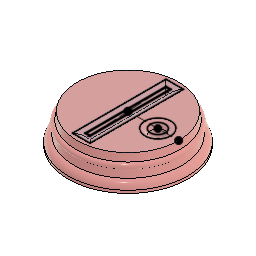
SoilSensorWaterProofCap (Autodesk Fusion 360 design; units mm, degrees)
Autodesk Fusion 360 part; units mm, degrees
note: some values were not read from the file. Set by a fixed rule: which face or edge a step refers to.
sketch "Sketch1" plane through (0, 0, 0) normal (0, 0, 1) x (1, 0, 0) in component "Cap"
  circle A0 centre (0, 0) radius 16.5
  circle A1 centre (0, 0) radius 14.9
  dimension "d1" = 33
  dimension "d2" = 29.8
  constraint coincident A0.centre A1.centre
  constraint concentric A0 A1
  measures "d1" diameter of A0
  measures "d2" diameter of A1
extrude "Extrude1" add sketch "Sketch1" along normal blind 2.5 makes body 1 in component "Cap"
sketch "Sketch2" plane through (0, 0, 2.5) normal (0, 0, 1) x (-1, 0, 0) in component "Cap"
  circle A0 centre (0, 0) radius 14.9
  circle A1 centre (0, 0) radius 16.5
  circle A2 centre (0, 0) radius 14.9
  constraint coincident A0.centre A1.centre
ref_plane "WorkPlane1" through (0, 0, 8) normal (0, 0, 1) x (1, 0, 0) in component "Cap"
sketch "Sketch3" plane through (0, 0, 8) normal (0, 0, 1) x (1, 0, 0) in component "Cap"
  circle A0 centre (0, 0) radius 14
  dimension "d6" = 28
  constraint coincident A0.centre origin
  measures "d6" diameter of A0
loft "Loft1" add profiles "Sketch3", "Sketch2" section 1 section 2 contours A0 A2 bodies 1 in component "Cap"
shell "Shell1" thickness 1 removed faces 1 at (0.561, -2.4191, 2.5) on bodies 1 in component "Cap"
ref_plane "WorkPlane2" through (0, 0, 5.25) normal (0, 0, 1) x (1, 0, 0) in component "Cap"
torus "TorusPrimitive1" add centre line diameter 29 section diameter 1.5 placed x (1, 0, 0) y (0, 1, 0) z (0, 0, 1) at (0, 0, 5.25) bodies 1 in component "Cap"
sketch "Sketch5" plane through (0, 0, 8) normal (0, 0, 1) x (-1, 0, 0) in component "Cap"
  circle A0 centre (0, 0) radius 14
sketch "Sketch6" plane through (0, 0, 8) normal (0, 0, 1) x (-1, 0, 0) in component "Cap"
  line L0 (0.7, -11.2) -> (-0.7, -11.2)
  line L1 (-0.7, -11.2) -> (-0.7, 11.2)
  line L2 (-0.7, 11.2) -> (0.7, 11.2)
  line L3 (0.7, 11.2) -> (0.7, -11.2)
  line L4 (0.7, -11.2) -> (-0.7, 11.2) construction
  line L5 (-2.4, -12.9) -> (-2.4, 12.9)
  line L6 (-2.4, 12.9) -> (2.4, 12.9)
  line L7 (2.4, 12.9) -> (2.4, -12.9)
  line L8 (2.4, -12.9) -> (-2.4, -12.9)
  line L9 (-0.5, -11) -> (-0.5, 11)
  line L10 (-0.5, 11) -> (0.5, 11)
  line L11 (0.5, 11) -> (0.5, -11)
  line L12 (0.5, -11) -> (-0.5, -11)
  dimension "d9" = 1.4
  dimension "d10" = 22.4
  dimension "d22" = -1.7
  dimension "d33" = 0.2
  constraint horizontal L0
  constraint vertical L1
  constraint horizontal L2
  constraint vertical L3
  constraint midpoint L4 origin
  measures "d9" distance of L0.start L0.end
  measures "d10" distance of L0.start L2.end
extrude "Extrude2" cut sketch "Sketch6" against normal up to surface (1 mm away) contours L0 L1 L2 L3 | L9 L10 L11 L12 bodies 1 in component "Cap"
extrude "Extrude3" add sketch "Sketch6" against normal up to surface (8 mm away) contours L5 L6 L7 L8 bodies 1 in component "Cap"
fillet "Fillet3" radius 1 4 edges at (2.4, 12.9, 3.5) (-2.4, 12.9, 3.5) (-2.4, -12.9, 3.5) (2.4, -12.9, 3.5) on bodies 1 in component "Cap"
extrude "Extrude4" add 1 faces at (14.5068, 0.7402, 2.5) along direction (0, 0, -1) blind 2.5 on bodies 1 bodies 1 in component "Cap"
extrude "Extrude5" add sketch "Sketch6" against normal blind 1 contours L0 L1 L2 L3 bodies 1 in component "Cap"
sketch "Sketch7" plane through (0, 0, 0) normal (0, 0, -1) x (1, 0, 0) in component "Cap"
  arc A0 (2.4, 11.9) -> (1.4, 12.9) centre (1.4, 11.9) ccw
  line L0 (1.4, 12.9) -> (-1.4, 12.9)
  arc A1 (-1.4, 12.9) -> (-2.4, 11.9) centre (-1.4, 11.9) ccw
  line L1 (-2.4, 11.9) -> (-2.4, -11.9)
  arc A2 (-2.4, -11.9) -> (-1.4, -12.9) centre (-1.4, -11.9) ccw
  line L2 (-1.4, -12.9) -> (1.4, -12.9)
  arc A3 (1.4, -12.9) -> (2.4, -11.9) centre (1.4, -11.9) ccw
  line L3 (2.4, -11.9) -> (2.4, 11.9)
  line L4 (-0.7, -11.2) -> (-0.7, 11.2)
  line L5 (-0.7, 11.2) -> (0.7, 11.2)
  line L6 (0.7, 11.2) -> (0.7, -11.2)
  line L7 (0.7, -11.2) -> (-0.7, -11.2)
  line L8 (0.5, -11) -> (0.5, 11)
  line L9 (0.5, 11) -> (-0.5, 11)
  line L10 (-0.5, 11) -> (-0.5, -11)
  line L11 (-0.5, -11) -> (0.5, -11)
  line L12 (0.7, -11.2) -> (0.7, 11.2)
  line L13 (0.7, 11.2) -> (-0.7, 11.2)
  line L14 (-0.7, -11.2) -> (0.7, -11.2)
  line L15 (-0.7, 11.2) -> (-0.7, -11.2)
extrude "Extrude6" add sketch "Sketch7" against normal blind 1 contours L4 L5 L6 L7 L12 L13 L14 L15 bodies 1 in component "Cap"
fillet "Fillet6" radius 2.5 4 edges at (0.5, 0, 8) (0, -11, 8) (-0.5, 0, 8) (0, 11, 8) on bodies 1 in component "Cap"
fillet "Fillet7" radius 2.5 4 edges at (-0.5, 0, 1) (0, -11, 1) (0.5, 0, 1) (0, 11, 1) on bodies 1 in component "Cap"
sketch "Sketch1 (2)" plane through (0, 0, 0) normal (0, 0, 1) x (1, 0, 0) in component "WireConnector"
  circle A0 centre (0, 0) radius 2
  circle A1 centre (0, 0) radius 9
  circle A2 centre (0, 0) radius 3
  dimension "d42" = 4
  dimension "d43" = 7
  dimension "d44" = 1
  constraint coincident A0.centre A1.centre
  measures "d42" diameter of A0
extrude "Extrude1'" add sketch "Sketch1 (2)" along normal blind 2 separate body contours A1 makes body 2 in component "WireConnector"
extrude "Extrude2'" add sketch "Sketch1 (2)" along normal blind 5 contours A2 bodies 2 in component "WireConnector"
fillet "Fillet1" radius 1 1 edges at (-2.797, -1.0848, 5) on bodies 2 in component "WireConnector"
sketch "Sketch2 (2)" plane through (0, 0, 2) normal (0, 0, 1) x (-1, 0, 0) in component "WireConnector"
  circle A0 centre (0, 0) radius 3
  circle A1 centre (0, 0) radius 9
  circle A2 centre (0, 0) radius 3
  circle A3 centre (0, 0) radius 2.5
  dimension "d51" = -0.5
extrude "Extrude3'" cut sketch "Sketch2 (2)" along normal blind 1 contours A0 A2 bodies 2 in component "WireConnector"
fillet "Fillet2" radius 0.5 1 edges at (2.3308, -0.904, 3) on bodies 2 in component "WireConnector"
sketch "Sketch1 (3)" plane through (0, 0, 0) normal (0, 0, 1) x (1, 0, 0) in component "WireTester"
  circle A0 centre (0, 0) radius 2.1
  circle A1 centre (0, 0) radius 4.1
  dimension "d56" = 4.2
  dimension "d57" = 2
  constraint coincident A0.centre A1.centre
  measures "d56" diameter of A0
sketch "Sketch8" plane through (0, 0, 8) normal (0, 0, 1) x (-1, 0, 0) in component "Cap"
  circle A0 centre (0, 0) radius 14
  line L0 (2.5, 13) -> (2.5, -13)
  line L1 (2.5, -13) -> (-2.5, -13)
  line L2 (-2.5, -13) -> (-2.5, 13)
  line L3 (-2.5, 13) -> (2.5, 13)
  line L4 (-2.5, 0) -> (-14, 0) construction
  circle A1 centre (-8.25, 0) radius 2.05
  circle A2 centre (-8.25, 0) radius 3.55
  point P0 (-14, 0)
  dimension "d64" = 4.1
  dimension "d69" = 1.5
  constraint midpoint L2 L4.start
  constraint coincident P0 L4.end
  constraint midpoint L4 A1.centre
  measures "d64" diameter of A1
extrude "Extrude7" cut sketch "Sketch8" against normal up to surface (1 mm away) contours A1 bodies 1 in component "Cap"
fillet "Fillet9" radius 1 1 edges at (10.1613, -0.7413, 8) on bodies 1 in component "Cap"
extrude "Extrude1''" add sketch "Sketch1 (3)" along normal blind 5 separate body makes body 3 in component "WireTester"
fillet "Fillet1'" radius 2 1 edges at (-1.9579, 0.7594, 5) on bodies 3 in component "WireTester"
fillet "Fillet8" radius 1.75 1 edges at (-15.3834, -5.9667, 2.5) on bodies 1 in component "Cap"
extrude "Extrude8" add sketch "Sketch8" against normal blind 5 contours A2 bodies 1 in component "Cap"
fillet "Fillet10" radius 1.5 1 edges at (10.1613, -0.7413, 8) on bodies 1 in component "Cap"
component "Cap" placed x (1, 0, 0) y (0, 1, 0) z (0, 0, 1) at (0, 0, 0)
component "WireConnector" placed x (1, 0, 0) y (0, 1, 0) z (0, 0, 1) at (0, 0, 0)
component "WireTester" placed x (1, 0, 0) y (0, 1, 0) z (0, 0, 1) at (0, 0, 0)
